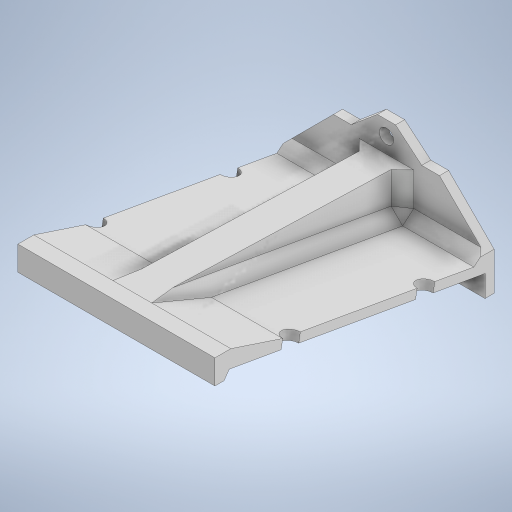
# Autodesk Inventor part: BreadboardHolder-v2
Saved by Autodesk Inventor 2023 (Build 270158030, 158C)
## iProperties
Created: 2024-03-25
Part Number: BreadboardHolder-v2
Material: Generic
Document SubType Name: Modeling
Designer: lvrectanus0
Density: 1 g/cm^3
Appearance: Default
Author: lvrectanus0
Autodesk Inventor part; units mm, degrees
ref_plane "YZ Plane" through (0, 0, 0) normal (1, 0, 0) x (0, 1, 0)
ref_plane "XZ Plane" through (0, 0, 0) normal (0, 1, 0) x (-1, 0, 0)
sketch "Sketch2" plane through (0, 0, 0) normal (1, 0, 0) x (0, 1, 0)
  line L0 (-23.6605, 0) -> (-23.6605, 2.54)
  line L1 (-23.6605, 2.54) -> (-17.3105, 2.54)
  line L2 (-17.3105, 2.54) -> (-4.721, 73.9386)
  line L3 (10.5271, 0) -> (9.3929, 0) projected
  line L4 (-4.721, 73.9386) -> (-2.2195, 73.4975)
  line L5 (-4.721, 73.9386) -> (-2.181, 73.9386) construction
  line L6 (-23.3526, 2.54) -> (0, 2.54)
  line L7 (0, 2.54) -> (0, 0)
  line L8 (0, 0) -> (-23.3526, 0)
  line L9 (-23.3526, 0) -> (-23.3526, 2.54)
  line L10 (-2.2195, 73.4975) -> (-14.7313, 2.54)
  point P0 (23.6605, 0)
  point P1 (-4.0951, 0)
  point P2 (-6.6351, 0)
  dimension "d2" = 2.54
  dimension "d3" = 6.35
  dimension "d5" = 100
  dimension "d6" = 2.54
  dimension "d7" = 10
  dimension "d9" = 72.5
  constraints: 20 end point, 3 parallel, 2 horizontal, 2 perpendicular, 2 point on line, 1 equal length, 1 vertical, 4 other
  measures "d2" distance of L0.start L0.end
  measures "d3" distance of L0.end L1.end
  measures "d5" angle of L2 L1
  measures "d6" distance of L2.end L4.end
  measures "d7" angle of L4 L5
  measures "d9" distance of L1.end L2.end
extrude "Extrusion1" add sketch "Sketch2" along normal mid plane 55
sketch "Sketch3" plane through (0, 0, 0) normal (1, 0, 0) x (0, 1, 0)
  line L0 (-2.2195, 73.4975) -> (-2.2195, 2.54)
  line L1 (0, 2.54) -> (-14.7313, 2.54) projected
  line L2 (-14.7313, 2.54) -> (-2.2195, 73.4975)
  line L3 (-2.2195, 73.4975) -> (-14.7313, 2.54) projected
  line L4 (-2.2195, 73.4975) -> (0, 73.4975)
  line L5 (0, 73.4975) -> (-2.2195, 2.54)
  point P0 (0, 0)
  constraints: 8 end point, 1 horizontal, 1 point on line, 1 vertical
extrude "Extrusion2" add sketch "Sketch3" along normal mid plane 8.89
sketch "Sketch4" plane through (-27.5, -17.3105, 2.54) normal (0, -0.9848078, 0.1736482) x (1, 0, 0)
  line L0 (2.5, 71.4739) -> (2.5, 1.4739) construction
  line L1 (2.5, 1.4739) -> (52.5, 1.4739) construction
  line L2 (52.5, 1.4739) -> (52.5, 71.4739) construction
  line L3 (52.5, 71.4739) -> (2.5, 71.4739) construction
  line L4 (2.5, 71.4739) -> (52.5, 1.4739) construction
  line L5 (2.5, 1.4739) -> (52.5, 71.4739) construction
  line L6 (55, 0.4479) -> (55, 72.5) projected
  line L7 (2.5, 71.4739) -> (72.5, 71.4739) construction
  line L8 (55, 36.4739) -> (55, 71.4739)
  line L9 (55, 36.4739) -> (55, 1.4739)
  line L10 (55, 72.5) -> (55, 0) projected
  line L11 (55, 55.3) -> (52.5, 55.3)
  line L12 (55, 17.2) -> (52.5, 17.2)
  line L13 (0, 0) -> (0, 72.5) projected
  line L14 (0, 36.4739) -> (0, 71.4739)
  line L15 (0, 36.4739) -> (0, 1.7269)
  line L16 (0, 0.4479) -> (0, 3.0059) projected
  line L17 (0, 17.2) -> (2.5, 17.2)
  line L18 (0, 55.3) -> (2.5, 55.3)
  circle A0 centre (55, 55.3) radius 2.5
  circle A1 centre (55, 17.2) radius 2.5
  circle A2 centre (0, 55.3) radius 2.5
  circle A3 centre (0, 17.2) radius 2.5
  point P0 (27.5, 0.5045)
  point P1 (27.5, 36.4739)
  point P2 (27.5, 36.4739)
  point P3 (27.5, 36.4739)
  point P4 (55, 36.25)
  point P5 (55, 36.25)
  point P6 (0, 52.8)
  point P7 (0, 57.8)
  point P8 (0, 14.7)
  point P9 (0, 19.7)
  point P10 (55, 14.7)
  point P11 (55, 19.7)
  point P12 (55, 52.8)
  point P13 (55, 57.8)
  dimension "d14" = 70
  dimension "d15" = 90
  dimension "d16" = 50
  dimension "d17" = 19.05
  dimension "d18" = 19.05
  constraints: 30 end point, 14 point on line, 6 midpoint, 4 coincident, 4 perpendicular, 3 parallel, 1 horizontal, 1 horizontal alignment, 1 vertical alignment, 18 other
  measures "d14" distance of L0.start L0.end
  measures "d15" angle of L0 L7
  measures "d16" distance of L1.end L0.end
  measures "d17" distance of point (55, 36.25) L11.start
  measures "d18" distance of L12.start point (55, 36.25)
extrude "Extrusion3" cut sketch "Sketch4" against normal through all contours A1 L12 L6 | L12 A1 L6 | A0 L11 L6 | L11 A0 L6 | L13 L17 A3 | L13 A3 L17 | L13 L18 A2 | L13 A2 L18
sketch "Sketch5" plane through (-27.5, 0, 2.54) normal (0, 0, 1) x (1, 0, 0)
  line L0 (64.0804, -22.4444) -> (30.0297, 6.1276) projected
  line L1 (-9.0804, -22.4444) -> (24.9703, 6.1276) projected
  line L2 (30.0297, 6.1276) -> (24.9703, 6.1276)
  line L3 (0, 0) -> (55, 0) projected
  line L4 (37.3323, 0) -> (17.6677, 0)
  point P0 (27.5, 0)
  constraints: 4 end point, 4 point on line, 1 horizontal
ref_plane "Work Plane1" through (-49.846, -23.6605, 0) normal (0, 0, 1) x (1, 0, 0)
extrude "Extrusion4" add sketch "Sketch5" against normal up to surface (2.54 mm away)
chamfer "Chamfer1" distance 12.7 angle 45 2 edges at (-27.5, 0, 1.27) (27.5, 0, 1.27)
sketch "Sketch6" plane through (-27.5, 0, 0) normal (-1, 0, 0) x (0, 0, 1)
  line L0 (73.9386, -4.721) -> (73.4975, -2.2195) projected
  line L1 (73.9386, -4.721) -> (75.3954, -6.8016)
  line L2 (73.9386, -4.721) -> (76.4786, -4.721) construction
  line L3 (75.3954, -6.8016) -> (75.3954, 0)
  line L4 (75.3954, 0) -> (73.4975, 0)
  line L5 (73.4975, 0) -> (73.4975, -2.2195)
  line L6 (54.0968, -5.6404) -> (59.0208, -4.7722) projected
  line L7 (73.4975, 0) -> (59.0208, -4.7722)
  line L8 (59.0208, -4.7722) -> (73.4975, -2.2195)
  line L9 (75.3954, -6.8016) -> (77.9354, -6.8016)
  line L10 (77.9354, -6.8016) -> (77.9354, 0)
  line L11 (77.9354, 0) -> (75.3954, 0)
  line L12 (75.3954, 0) -> (75.3954, -6.8016)
  point P0 (0, 0)
  dimension "d26" = 2.54
  dimension "d27" = 55
  dimension "d30" = 2.54
  constraints: 22 end point, 3 perpendicular, 2 horizontal, 2 parallel, 1 collinear, 1 equal length, 1 horizontal alignment, 1 vertical
  measures "d26" distance of L0.start L1.end
  measures "d27" angle of L1 L2
  measures "d30" distance of L11.end L10.end
extrude "Extrusion5" add sketch "Sketch6" against normal up to surface (55 mm away)
sketch "Sketch7" plane through (-27.5, -14.7313, 2.54) normal (0, 0, 1) x (1, 0, 0)
  line L0 (12.7, 14.7313) -> (17.6677, 14.7313) construction
  line L1 (37.3323, 14.7313) -> (17.6677, 14.7313) construction
  line L2 (27.5, 14.7313) -> (27.5, 20.8588) construction
  line L3 (30.0297, 20.8588) -> (24.9703, 20.8588) construction
  line L4 (0, -2.5792) -> (55, -2.5792) construction
  line L5 (0, 2.0313) -> (0, -8.6214) construction
  line L6 (55, -2.5792) -> (0, -8.6214) construction
  line L7 (0, -8.6214) -> (0, -2.5792) construction
  line L8 (0, -8.6214) -> (55, -8.6214) construction
  line L9 (55, -8.6214) -> (0, -2.5792) construction
  line L10 (55, -8.6214) -> (55, 2.0313) construction
  line L11 (55, -5.6003) -> (0, -5.6003) construction
  point P0 (27.5, 16.8588)
  point P1 (40.2, -5.6003)
  point P2 (14.8, -5.6003)
  point P3 (27.5, -5.6003)
  point P4 (27.5, -5.6003)
  dimension "d31" = 4
  dimension "d39" = 12.7
  dimension "d40" = 12.7
  constraints: 12 end point, 5 point on line, 4 midpoint, 1 collinear
  measures "d31" distance from line of point (27.5, 16.859) L3
  measures "d39" distance of point (27.5, -5.6) point (40.2, -5.6)
  measures "d40" distance of point (14.8, -5.6) point (27.5, -5.6)
hole "Hole1" at (0, 2.1276, 2.54) at (12.7, -20.3315, 2.54) at (-12.7, -20.3315, 2.54) direction (0, 0, -1) diameter 4 depth 5.8
chamfer "Chamfer2" distance 3.175 angle 45 6 edges at (4.445, -9.7517, 30.7804) (15.9725, -14.7313, 2.54) (-4.445, -9.7517, 30.7804) (-15.9725, -14.7313, 2.54) (-4.445, -8.4754, 2.54) (4.445, -8.4754, 2.54)
body "Solid1"
